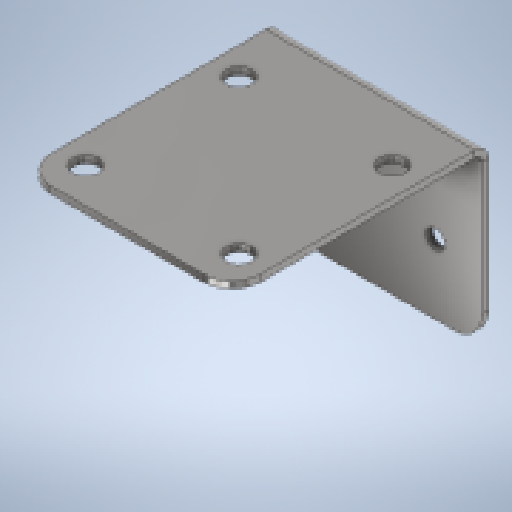
# Autodesk Inventor part: 2309HCMUTE-CDT23-DO_GA
Saved by Autodesk Inventor 2023 (Build 270158000, 158)
## iProperties
Created: 2023-10-15
Part Number: 2309HCMUTE-CDT23-DO_GA
Material: Stainless Steel
Document SubType Name: Sheet Metal
Designer: havie
Density: 8 g/cm^3
Sheet Metal Rule: Default_mm
Appearance: Steel - Polished
Author: havie
Autodesk Inventor part; units mm, degrees
ref_plane "YZ Plane" through (0, 0, 0) normal (1, 0, 0) x (0, 1, 0)
ref_plane "XZ Plane" through (0, 0, 0) normal (0, 1, 0) x (-1, 0, 0)
ref_plane "XY Plane" through (0, 0, 0) normal (0, 0, 1) x (1, 0, 0)
sketch "Sketch1" plane through (0, 0, 0) normal (0, 0, 1) x (1, 0, 0)
  line L0 (-22.5, 45) -> (22.5, 45)
  line L1 (22.5, 45) -> (22.5, -45)
  line L2 (22.5, -45) -> (-22.5, -45)
  line L3 (-22.5, -45) -> (-22.5, 45)
  line L4 (-22.5, 45) -> (22.5, -45) construction
  line L5 (22.5, 45) -> (-22.5, -45) construction
  point P0 (0, 0)
  dimension "d0" = 90
  dimension "d1" = 45
  measures "d0" distance of L0.end L1.end
  measures "d1" distance of L0.start L0.end
extrude "Plate1" add sketch "Sketch1" along normal mid plane 1.5
sketch "Sketch2" plane through (0, 0, 0.75) normal (0, 0, 1) x (1, 0, 0)
  line L0 (-22.5, -45) -> (-22.5, 45) projected
  line L1 (-22.5, -9) -> (22.5, -9)
  line L2 (-22.5, 45) -> (22.5, 45) projected
  line L3 (22.5, 45) -> (22.5, -45) projected
  point P0 (0, 0)
  dimension "d3" = 54
  constraints: 2 end point, 2 point on line, 1 horizontal
  measures "d3" distance between parallel lines of L2 L1
fold "Fold1" angle 90 bend radius 1.5 thickness 1.5 k factor 0.44 line from (-22.5, -9, 0.75) to (22.5, -9, 0.75) line at bend centre moving side (0, 1, 0) folds toward (0, 0, 1)
sketch "Sketch3" plane through (-22.5, -9.1965, 54.5535) normal (0, -1, 0) x (1, 0, 0)
  line L0 (0, 0) -> (45, 0) projected
  line L1 (0, -52.3035) -> (0, 0) projected
  point P0 (22.5, -54.5535)
  point P1 (6, -7.5)
  point P2 (39, -7.5)
  point P3 (39, -40.5)
  point P4 (6, -40.5)
  dimension "d10" = 7.5
  dimension "d11" = 33
  dimension "d12" = 33
  dimension "d13" = 6
  constraints: 2 horizontal alignment, 2 vertical alignment
  measures "d10" distance from line of L0 point (6, -7.5)
  measures "d11" distance of point (6, -40.5) point (6, -7.5)
  measures "d12" distance of point (39, -7.5) point (6, -7.5)
  measures "d13" distance from line of L1 point (6, -7.5)
hole "Hole1" at (-16.5, -9.1965, 47.0535) at (16.5, -9.1965, 47.0535) at (16.5, -9.1965, 14.0535) at (-16.5, -9.1965, 14.0535) direction (0, 1, 0) diameter 5.5 end through all
fillet "Corner Round1" radius 6 2 edges at (-22.5, -8.4465, 54.5535) (22.5, -8.4465, 54.5535)
sketch "Sketch4" plane through (0, 0, 0.75) normal (0, 0, 1) x (1, 0, 0)
  line L0 (22.5, -45) -> (-22.5, -45) projected
  line L1 (22.5, -10.6965) -> (22.5, -45) projected
  line L2 (-22.5, -45) -> (-22.5, -10.6965) projected
  point P0 (0, 0)
  point P1 (12.5, -30)
  point P2 (-12.5, -30)
  dimension "d22" = 15
  dimension "d23" = 10
  dimension "d24" = 10
  constraints: 1 horizontal alignment
  measures "d22" distance from line of L0 point (12.5, -30)
  measures "d23" distance from line of L1 point (12.5, -30)
  measures "d24" distance from line of L2 point (-12.5, -30)
hole "Hole2" at (12.5, -30, 0.75) at (-12.5, -30, 0.75) direction (0, 0, -1) diameter 5.5 end through all
fillet "Corner Round2" radius 6 2 edges at (-22.5, -45, 0) (22.5, -45, 0)
equation "\"d2\" = Thickness"
equation "\"d4\" = BendReliefWidth"
equation "\"d5\" = BendReliefDepth"
equation "\"d6\" = MinimumRemnant"
equation "\"d7\" = TransitionRadius"
equation "\"d9\" = BendRadius"
equation "\"d19\" = Thickness"
equation "\"BendRadius\" = Thickness"
equation "\"BendReliefWidth\" = Thickness"
equation "\"BendReliefDepth\" = 0.5 * Thickness"
equation "\"CornerReliefSize\" = 4 * Thickness"
equation "\"MinimumRemnant\" = 2 * Thickness"
equation "\"TransitionRadius\" = BendRadius"
equation "\"JacobiRadiusSize\" = BendRadius"
equation "\"GapSize\" = Thickness"
equation "\"Thickness\" = 1.5"
body "Solid1"
